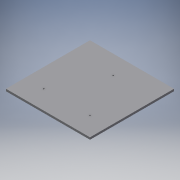
# Autodesk Inventor part: Base
Saved by Autodesk Inventor 2016 (Build 200138000, 138)
## iProperties
Created: 2017-05-15
Part Number: Base
Material: Generic
Document SubType Name: Modeling
Designer: 31745
Density: 1 g/cm^3
Appearance: Default
Author: 31745
Autodesk Inventor part; units mm, degrees
ref_plane "YZ Plane" through (0, 0, 0) normal (1, 0, 0) x (0, 1, 0)
ref_plane "XZ Plane" through (0, 0, 0) normal (0, 1, 0) x (-1, 0, 0)
ref_plane "XY Plane" through (0, 0, 0) normal (0, 0, 1) x (1, 0, 0)
sketch "Sketch1" plane through (0, 0, 0) normal (0, 1, 0) x (-1, 0, 0)
  line L0 (0, 0) -> (-254, 0)
  line L1 (-254, 0) -> (-254, -254)
  line L2 (-254, -254) -> (0, -254)
  line L3 (0, -254) -> (0, 0)
  dimension "d0" = 254
  dimension "d1" = 254
  constraints: 8 end point, 2 parallel, 1 horizontal, 1 perpendicular
  measures "d0" distance of L2.end L1.end
  measures "d1" distance of L1.end L0.end
extrude "Extrusion1" add sketch "Sketch1" along normal blind 6.35
sketch "Sketch2" plane through (0, 6.35, 0) normal (0, 1, 0) x (1, 0, 0)
  line L0 (254, 254) -> (0, 254) projected
  line L1 (127, 196.85) -> (127, 57.15)
  line L2 (127, 57.15) -> (57.15, 57.15)
  line L3 (57.15, 57.15) -> (196.85, 57.15)
  line L4 (0, 254) -> (0, 0) projected
  point P0 (127, 254)
  point P1 (127, 127)
  point P2 (0, 127)
  dimension "d4" = 69.85
  dimension "d5" = 69.85
  dimension "d6" = 139.7
  constraints: 6 end point, 3 midpoint, 2 horizontal alignment, 1 collinear, 1 perpendicular, 1 vertical, 1 vertical alignment
  measures "d4" horizontal distance of L1.start L2.end
  measures "d5" horizontal distance of L3.end L1.start
  measures "d6" vertical distance of L2.end L1.start
hole "Hole1" at (57.15, 6.35, -57.15) at (196.85, 6.35, -57.15) at (127, 6.35, -196.85) direction (0, -1, 0) diameter 3.302 end through all thread size "8-32 UNC" class "2B" standard "ANSI Unified Screw Threads"
equation "\"d5\" = d4"
body "Solid1"
